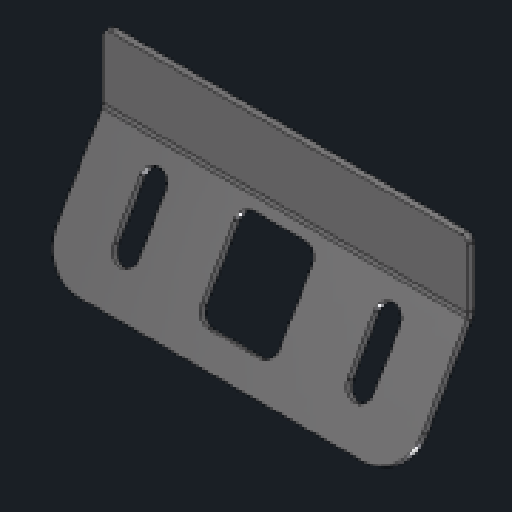
# Autodesk Inventor part: Model-4_Sheet Stifferner
Saved by Autodesk Inventor 2025.1 (Build 291241000, 241)
## iProperties
RuleStatus: InUse
Created: 2026-02-13
Part Number: Model-4_Sheet Stifferner
User Status: Released
Material: SS304
Document SubType Name: Sheet Metal
Designer: Desktop -24
Density: 7.99949 g/cm^3
Sheet Metal Rule: 1/4"
Appearance: Semi-Polished(1)
AfterDocNew0: Mat. Selection
encoded128: ÌSheet Metal (in)XÎ
Family: SS304
Author: Desktop -24
Revision Number: 0
Autodesk Inventor part; units mm, degrees
ref_plane "YZ Plane" through (0, 0, 0) normal (1, 0, 0) x (0, 1, 0)
ref_plane "XZ Plane" through (0, 0, 0) normal (0, 1, 0) x (-1, 0, 0)
ref_plane "XY Plane" through (0, 0, 0) normal (0, 0, 1) x (1, 0, 0)
sketch "Sketch1" plane through (0, 0, 0) normal (0, 0, 1) x (1, 0, 0)
  line L0 (-177.8, -31.75) -> (177.8, -31.75)
  line L1 (177.8, -31.75) -> (177.8, 31.75)
  line L2 (177.8, 31.75) -> (-177.8, 31.75)
  line L3 (-177.8, 31.75) -> (-177.8, -31.75)
  line L4 (-177.8, -31.75) -> (177.8, 31.75) construction
  line L5 (177.8, -31.75) -> (-177.8, 31.75) construction
  point P0 (0, 0)
  point P1 (0, 0)
  dimension "d31" = 355.6
  dimension "d32" = 63.5
  measures "d31" distance of L1.end L2.end
  measures "d32" distance of L0.end L1.end
extrude "Plate1" add sketch "Sketch1" along normal blind 6.35
sketch "Sketch3" plane through (177.8, -37.3716, 8.6786) normal (0, -0.7071068, -0.7071068) x (1, 0, 0)
  line L0 (-355.6, 0) -> (0, 0)
  line L1 (0, 0) -> (0, 150.7998)
  line L2 (0, 150.7998) -> (-355.6, 150.7998)
  line L3 (-355.6, 150.7998) -> (-355.6, 0)
  constraints: 6 end point, 1 horizontal, 1 perpendicular, 1 vertical
edge flange "Flange2" height 165.1 angle 45 thickness 6.35 bend radius 7.9502 thickness toward (0, -0.7071068, -0.7071068) relief tear relief width 6.35 relief depth 3.175 edges at (0, -31.75, 6.35) wall of the first edge with corners at (-177.8, -37.3716, 8.6786) (177.8, -37.3716, 8.6786) (177.8, -144.0032, 115.3101) (-177.8, -144.0032, 115.3101)
bend "Bend2"
corner "Corner2"
fillet "Corner Round1" radius 6.35 2 edges at (177.8, 31.75, 3.175) (-177.8, 31.75, 3.175)
fillet "Corner Round2" radius 38.1 2 edges at (177.8, -146.2483, 113.0651) (-177.8, -146.2483, 113.0651)
sketch "Sketch4" plane through (-177.8, -37.3716, 8.6786) normal (0, 0.7071068, 0.7071068) x (1, 0, 0)
  line L0 (152.4, -17.4498) -> (203.2, -17.4498)
  line L1 (215.9, -30.1498) -> (215.9, -115.8748)
  line L2 (203.2, -128.5748) -> (152.4, -128.5748)
  line L3 (139.7, -115.8748) -> (139.7, -30.1498)
  line L4 (139.7, -17.4498) -> (215.9, -128.5748) construction
  line L5 (215.9, -17.4498) -> (139.7, -128.5748) construction
  line L6 (38.1, -150.7998) -> (317.5, -150.7998) construction
  arc A0 (152.4, -17.4498) -> (139.7, -30.1498) centre (152.4, -30.1498) ccw
  arc A1 (215.9, -30.1498) -> (203.2, -17.4498) centre (203.2, -30.1498) ccw
  arc A2 (203.2, -128.5748) -> (215.9, -115.8748) centre (203.2, -115.8748) ccw
  arc A3 (139.7, -115.8748) -> (152.4, -128.5748) centre (152.4, -115.8748) ccw
  line L7 (63.5, -98.4123) -> (63.5, -47.6123) construction
  line L8 (50.8, -98.4123) -> (50.8, -47.6123)
  line L9 (76.2, -47.6123) -> (76.2, -98.4123)
  arc A4 (50.8, -98.4123) -> (76.2, -98.4123) centre (63.5, -98.4123) ccw
  arc A5 (76.2, -47.6123) -> (50.8, -47.6123) centre (63.5, -47.6123) ccw
  line L10 (0, -112.6998) -> (0, 0) projected
  line L11 (177.8, -73.0123) -> (177.8, -150.7998) construction
  line L12 (292.1, -98.4123) -> (292.1, -47.6123) construction
  line L13 (304.8, -98.4123) -> (304.8, -47.6123)
  line L14 (279.4, -47.6123) -> (279.4, -98.4123)
  arc A6 (279.4, -98.4123) -> (304.8, -98.4123) centre (292.1, -98.4123) ccw
  arc A7 (304.8, -47.6123) -> (279.4, -47.6123) centre (292.1, -47.6123) ccw
  point P0 (63.5, -73.0123)
  dimension "d45" = 22.225
  dimension "d46" = 76.2
  dimension "d47" = 111.125
  dimension "d50" = 12.7
  dimension "d51" = 12.7
  dimension "d52" = 50.8
  dimension "d53" = 63.5
  dimension "d54" = 25.4
  constraints: 30 end point, 16 point on circle, 12 tangent, 8 centre point, 8 point on line, 6 symmetric about line, 4 midpoint, 3 parallel, 2 equal radius, 2 vertical, 1 horizontal, 1 horizontal alignment, 1 perpendicular, 1 vertical alignment, 2 other
  measures "d45" distance between parallel lines of L2 L6
  measures "d46" distance of L4.end L5.end
  measures "d47" distance of L5.end L4.start
  measures "d50" radius of A0
  measures "d51" radius of A1
  measures "d52" distance of L8.start L8.end
  measures "d53" distance between parallel lines of L10 L7
  measures "d54" distance between parallel lines of L9 L8
extrude "Cut1" cut sketch "Sketch4" against normal blind 6.35
equation "\"d48\" = Thickness"
equation "\"d15\" = Thickness"
equation "\"d33\" = BendReliefWidth"
equation "\"d34\" = BendReliefDepth"
equation "\"d35\" = MinimumRemnant"
equation "\"d36\" = TransitionRadius"
equation "\"d39\" = BendRadius"
equation "\"d40\" = CornerReliefSize"
equation "\"d41\" = GapSize"
equation "\"d42\" = JacobiRadiusSize"
equation "\"BendReliefWidth\" = Thickness"
equation "\"BendReliefDepth\" = 0.5 * Thickness"
equation "\"CornerReliefSize\" = 4 * Thickness"
equation "\"MinimumRemnant\" = 2 * Thickness"
equation "\"TransitionRadius\" = BendRadius"
equation "\"JacobiRadiusSize\" = Thickness"
equation "\"GapSize\" = Thickness"
equation "\"Thickness\" = 6.35"
equation "\"BendRadius\" = 7.9502"
body "Solid1"
